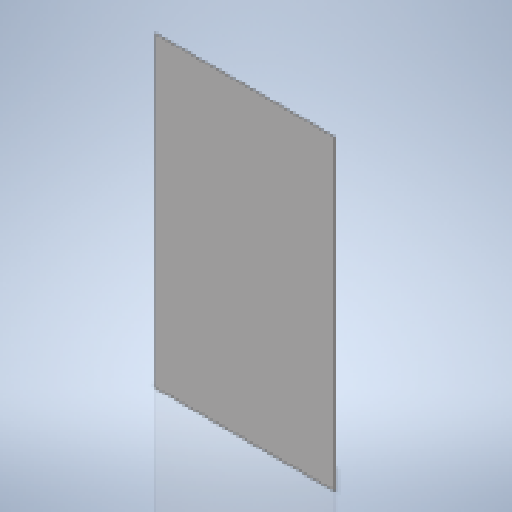
# Autodesk Inventor part: suporte_placa
Saved by Autodesk Inventor 2024.3 (Build 283343000, 343)
## iProperties
Created: 2024-06-28
Part Number: suporte_placa
Material: Genérico
Document SubType Name: Modeling
Designer: joaov
Density: 1 g/cm^3
Appearance: Padrão
Author: joaov
Autodesk Inventor part; units mm, degrees
ref_plane "YZ Plane" through (0, 0, 0) normal (1, 0, 0) x (0, 1, 0)
ref_plane "XZ Plane" through (0, 0, 0) normal (0, 1, 0) x (-1, 0, 0)
ref_plane "XY Plane" through (0, 0, 0) normal (0, 0, 1) x (1, 0, 0)
sketch "Esboço1" plane through (0, 0, 0) normal (0, 0, 1) x (1, 0, 0)
  line L0 (66.9586, -53.8463) -> (66.9586, -18.5463)
  line L1 (66.9586, -18.5463) -> (46.3396, -18.5463)
  line L2 (46.3396, -18.5463) -> (46.3396, -53.8463)
  line L3 (46.3396, -53.8463) -> (66.9586, -53.8463)
  point P0 (0, 0)
  dimension "d0" = 35.3
  dimension "d1" = 20.619
  constraints: 8 end point, 3 perpendicular, 1 vertical
  measures "d0" distance of L0.start L0.end
  measures "d1" distance of L0.end L1.end
extrude "Extrusão1" add sketch "Esboço1" along normal blind 2.5
chamfer "Chanfro1" distance 2.5 angle 45 2 edges at (56.6491, -18.5463, 0) (66.9586, -36.1963, 0)
sketch "Esboço2" plane through (0, 0, 2.5) normal (0, 0, 1) x (1, 0, 0)
  line L0 (66.9586, -18.5463) -> (46.3396, -18.5463) projected
  line L1 (46.3396, -18.5463) -> (46.3396, -11.6463)
  line L2 (46.3396, -11.6463) -> (66.9586, -11.6463)
  line L3 (66.9586, -11.6463) -> (66.9586, -18.5463)
  line L4 (66.9586, -18.5463) -> (46.3396, -18.5463)
  line L5 (46.3396, -18.5463) -> (46.3396, -19.5463)
  line L6 (46.3396, -19.5463) -> (66.9586, -19.5463)
  line L7 (66.9586, -19.5463) -> (66.9586, -18.5463)
  point P0 (0, 0)
  dimension "d7" = 6.9
  dimension "d10" = 1
  constraints: 14 end point, 5 perpendicular, 1 collinear, 1 vertical
  measures "d7" distance of L0.end L1.end
  measures "d10" distance of L0.end L5.end
extrude "Extrusão2" add sketch "Esboço2" along normal blind 2.5
chamfer "Chanfro2" distance 2.5 angle 45 1 edges at (56.6491, -19.5463, 2.5)
